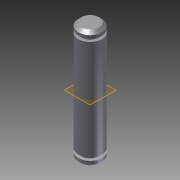
# Autodesk Inventor part: TU-010
Saved by Autodesk Inventor 2011 (Build 150229000, 229)
## iProperties
Shininess: 64.0
Angle Display Precision: 2
Document Length Units: 11269
Document Angle Units: 11279
Document Time Units: 11290
Document Mass Units: 11286
Document Length Units Precision: 3
Document Angle Units Precision: 2
Compacted: True
Created: 2002-07-24
Part Number: TU-010
Document SubType Name: Modeling
Designer: PN
Description: Short Pin
Density: 1 g/cm^3
Mass: 1.9436 g
Surface Area: 11.4919 cm^2
Volume: 1.9436 cm^3
Density: 0.0
Volumn: 0.0
Area: 0.0
PropertySet Name: Model Information
Control State: 0
Master: False
Checked Out: False
LENGTH: 1.000 in
Author: PN
Autodesk Inventor part; units mm, degrees
ref_plane "YZ Plane" through (0, 0, 0) normal (1, 0, 0) x (0, 1, 0)
ref_plane "XY Plane" through (0, 0, 0) normal (0, 0, 1) x (1, 0, 0)
sketch "Sketch1" plane through (0, 0, 0) normal (0, 0, 1) x (1, 0, 0)
  line L0 (3, 17) -> (4, 17)
  line L1 (4, 17) -> (4, -17)
  line L2 (4, -17) -> (3, -17)
  line L3 (3, -17) -> (3, -18)
  line L4 (3, -18) -> (4, -18)
  line L5 (4, -18) -> (4, -19)
  line L6 (4, -19) -> (3, -20)
  line L7 (0, 20) -> (3, 20)
  line L8 (3, 20) -> (4, 19)
  line L9 (4, 19) -> (4, 18)
  line L10 (4, 18) -> (3, 18)
  line L11 (3, 18) -> (3, 17)
  line L12 (0, 20) -> (0, -20)
  line L13 (0, -20) -> (3, -20)
  point P0 (0, 0)
  dimension "d4" = 35
  dimension "d5" = 1
  dimension "d6" = 36
  dimension "d7" = 2
  constraints: 28 end point, 6 parallel, 5 perpendicular, 1 horizontal, 1 midpoint, 1 vertical
  measures "d4" distance between parallel lines of L10 L2
  measures "d5" distance between parallel lines of L10 L0
  measures "d6" distance between parallel lines of L10 L4
  measures "d7" distance between parallel lines of L10 L7
revolve "Revolution1" add sketch "Sketch1" angle 360 about axis through (0, 20, 0) along (0, -1, 0)
equation "\"LENGTH\" = 25.4"
body "Solid1"
